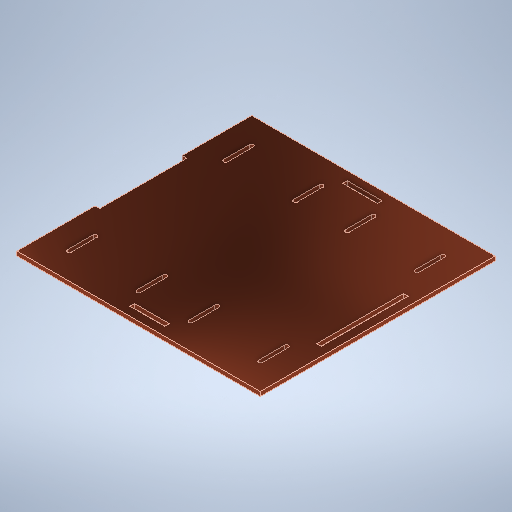
# Autodesk Inventor part: base_2
Saved by Autodesk Inventor 2025.3 (Build 293356030, 356C)
## iProperties
Created: 2026-06-26
Part Number: base_2
Material: Generic
Document SubType Name: Modeling
Designer: user
Density: 1 g/cm^3
Appearance: Copper - Polished
Author: user
Autodesk Inventor part; units mm, degrees
ref_plane "YZ Plane" through (0, 0, 0) normal (1, 0, 0) x (0, 1, 0)
ref_plane "XZ Plane" through (0, 0, 0) normal (0, 1, 0) x (-1, 0, 0)
ref_plane "XY Plane" through (0, 0, 0) normal (0, 0, 1) x (1, 0, 0)
sketch "Sketch1" plane through (0, 0, 0) normal (0, 1, 0) x (-1, 0, 0)
  line L0 (0, 0) -> (-280, 0)
  line L1 (-280, 0) -> (-280, -270)
  line L2 (-280, -270) -> (0, -270)
  line L3 (0, -270) -> (0, 0)
  line L4 (0, -135) -> (-280, -135) construction
  line L5 (-140, 0) -> (-140, -270) construction
  line L6 (-70, 0) -> (-70, -270) construction
  line L7 (-210, 0) -> (-210, -270) construction
  line L8 (-30, -240) -> (-30, -210) construction
  line L9 (-30, -240) -> (-30, -210) construction
  line L10 (-27.75, -240) -> (-27.75, -210)
  line L11 (-32.25, -210) -> (-32.25, -240)
  arc A0 (-32.25, -240) -> (-27.75, -240) centre (-30, -240) ccw
  arc A1 (-27.75, -210) -> (-32.25, -210) centre (-30, -210) ccw
  line L12 (-110, -240) -> (-110, -210) construction
  line L13 (-110, -240) -> (-110, -210) construction
  line L14 (-112.25, -240) -> (-112.25, -210)
  line L15 (-107.75, -210) -> (-107.75, -240)
  arc A2 (-112.25, -240) -> (-107.75, -240) centre (-110, -240) ccw
  arc A3 (-107.75, -210) -> (-112.25, -210) centre (-110, -210) ccw
  line L16 (-160, -260) -> (-120, -260)
  line L17 (-120, -260) -> (-120, -254.7)
  line L18 (-120, -254.7) -> (-160, -254.7)
  line L19 (-160, -254.7) -> (-160, -260)
  line L20 (-250, -240) -> (-250, -210) construction
  line L21 (-250, -240) -> (-250, -210) construction
  line L22 (-252.25, -240) -> (-252.25, -210)
  line L23 (-247.75, -210) -> (-247.75, -240)
  arc A4 (-252.25, -240) -> (-247.75, -240) centre (-250, -240) ccw
  arc A5 (-247.75, -210) -> (-252.25, -210) centre (-250, -210) ccw
  line L24 (-172.25, -210) -> (-172.25, -240)
  line L25 (-170, -240) -> (-170, -210) construction
  line L26 (-167.75, -240) -> (-167.75, -210)
  arc A6 (-172.25, -240) -> (-167.75, -240) centre (-170, -240) ccw
  line L27 (-170, -240) -> (-170, -210) construction
  arc A7 (-167.75, -210) -> (-172.25, -210) centre (-170, -210) ccw
  line L28 (-140, -270) -> (-140, 0) construction
  line L29 (-30, -30) -> (-30, -60) construction
  line L30 (-30, -30) -> (-30, -60) construction
  line L31 (-27.75, -30) -> (-27.75, -60)
  line L32 (-32.25, -60) -> (-32.25, -30)
  arc A8 (-27.75, -30) -> (-32.25, -30) centre (-30, -30) ccw
  arc A9 (-32.25, -60) -> (-27.75, -60) centre (-30, -60) ccw
  line L33 (-107.75, -60) -> (-107.75, -30)
  line L34 (-110, -30) -> (-110, -60) construction
  line L35 (-112.25, -30) -> (-112.25, -60)
  arc A10 (-107.75, -30) -> (-112.25, -30) centre (-110, -30) ccw
  line L36 (-110, -30) -> (-110, -60) construction
  arc A11 (-112.25, -60) -> (-107.75, -60) centre (-110, -60) ccw
  line L37 (-160, -10) -> (-120, -10)
  line L38 (-120, -10) -> (-120, -15.3)
  line L39 (-120, -15.3) -> (-160, -15.3)
  line L40 (-160, -15.3) -> (-160, -10)
  arc A12 (-247.75, -30) -> (-252.25, -30) centre (-250, -30) ccw
  line L41 (-247.75, -60) -> (-247.75, -30)
  line L42 (-250, -30) -> (-250, -60) construction
  line L43 (-250, -30) -> (-250, -60) construction
  arc A13 (-252.25, -60) -> (-247.75, -60) centre (-250, -60) ccw
  line L44 (-252.25, -30) -> (-252.25, -60)
  line L45 (-172.25, -60) -> (-172.25, -30)
  line L46 (-170, -30) -> (-170, -60) construction
  line L47 (-170, -30) -> (-170, -60) construction
  arc A14 (-172.25, -60) -> (-167.75, -60) centre (-170, -60) ccw
  line L48 (-167.75, -30) -> (-167.75, -60)
  arc A15 (-167.75, -30) -> (-172.25, -30) centre (-170, -30) ccw
  line L49 (-270, -95) -> (-270, -145)
  line L50 (-270, -145) -> (-270, -180)
  line L51 (-270, -180) -> (-264.7, -180)
  line L52 (-264.7, -180) -> (-264.7, -80)
  line L53 (-264.7, -80) -> (-270, -80)
  line L54 (-270, -80) -> (-270, -95)
  line L55 (0, -90) -> (-5.3, -90)
  line L56 (-5.3, -90) -> (-5.3, -190)
  line L57 (-5.3, -190) -> (0, -190)
  line L58 (0, -190) -> (0, -90)
  point P0 (-30, -225)
  point P1 (-110, -225)
  point P2 (-250, -225)
  point P3 (-170, -225)
  point P4 (-30, -45)
  point P5 (-110, -45)
  point P6 (-250, -45)
  point P7 (-170, -45)
  point P8 (0, -190)
  dimension "d0" = 280
  dimension "d1" = 270
  dimension "d2" = 30
  dimension "d3" = 40
  dimension "d4" = 30
  dimension "d6" = 2.25
  dimension "d9" = 40
  dimension "d13" = 10
  dimension "d14" = 5.3
  dimension "d16" = 20
  dimension "d20" = 10
  dimension "d21" = 5.3
  dimension "d22" = 5.3
  constraints: 134 end point, 55 symmetric about line, 32 point on circle, 16 centre point, 8 equal length, 6 point on line, 5 midpoint, 5 perpendicular, 4 tangent, 3 horizontal, 1 vertical, 14 other
  measures "d0" distance of L2.end L1.end
  measures "d1" distance of L1.end L0.end
  measures "d2" distance of L8.start L8.end
  measures "d3" distance between parallel lines of L6 L8
  measures "d4" distance from line of L2 L8.start
  measures "d6" radius of A0
  measures "d9" distance of L18.end L17.end
  measures "d13" distance between parallel lines of L2 L16
  measures "d14" distance between parallel lines of L18 L16
  measures "d16" distance between parallel lines of L5 L19
  measures "d20" distance between parallel lines of L1 L50
  measures "d21" distance of L57.end L56.end
  measures "d22" distance between parallel lines of L50 L52
extrude "Extrusion1" add sketch "Sketch1" along normal blind 5 contours L3 L55 L56 L57 L2 L1 L0
body "Solid1"
